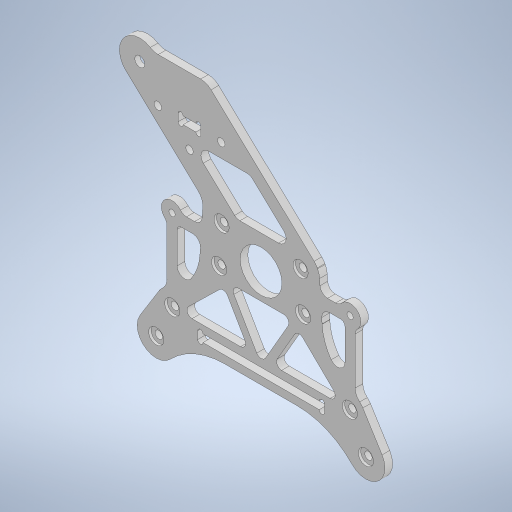
# Autodesk Inventor part: 内中間ユニット
Saved by Autodesk Inventor 2023 (Build 270158000, 158)
## iProperties
Created: 2022-06-23
Part Number: 内中間ユニット
Material: 一般
Document SubType Name: Modeling
Designer: muzho
Density: 1 g/cm^3
Appearance: 既定
Author: muzho
Autodesk Inventor part; units mm, degrees
ref_plane "YZ Plane" through (0, 0, 0) normal (1, 0, 0) x (0, 1, 0)
ref_plane "XZ Plane" through (0, 0, 0) normal (0, 1, 0) x (-1, 0, 0)
ref_plane "XY Plane" through (0, 0, 0) normal (0, 0, 1) x (1, 0, 0)
sketch "スケッチ1" plane through (0, 0, 0) normal (0, 0, 1) x (1, 0, 0)
  arc A0 (10.8616, 68.6715) -> (8.806, 69.4865) centre (8.806, 66.4865) ccw
  line L0 (10.8616, 68.6715) -> (23.2169, 57.0481)
  arc A1 (21.1613, 51.863) -> (23.2169, 57.0481) centre (21.1613, 54.863) ccw
  line L1 (21.1613, 51.863) -> (5.9002, 51.863)
  arc A2 (3.8446, 52.678) -> (5.9002, 51.863) centre (5.9002, 54.863) ccw
  line L2 (3.8446, 52.678) -> (-8.5107, 64.3014)
  arc A3 (-6.4551, 69.4865) -> (-8.5107, 64.3014) centre (-6.4551, 66.4865) ccw
  line L3 (-6.4551, 69.4865) -> (8.806, 69.4865)
  circle A4 centre (-1.4497, 74.9865) radius 1.5
  line L4 (35.1785, 52.6598) -> (-5.4497, 90.8816)
  arc A5 (-5.4497, 90.8816) -> (-9.561, 92.5115) centre (-9.561, 86.5115) ccw
  line L5 (-9.561, 92.5115) -> (-26.2964, 92.5115)
  arc A6 (-29.402, 93.3778) -> (-26.2964, 92.5115) centre (-26.2964, 98.5115) ccw
  arc A7 (-29.402, 93.3778) -> (-39.0547, 80.6665) centre (-33.5559, 86.5115) ccw
  line L6 (-39.0547, 80.6665) -> (-10.5496, 53.8498)
  arc A8 (-8.7348, 48.5407) -> (-10.5496, 53.8498) centre (-14.6609, 49.4798) ccw
  arc A9 (-8.7348, 48.5407) -> (-8.8114, 47.856) centre (-1.3025, 47.363) ccw
  line L7 (-8.9682, 45.4678) -> (-8.8114, 47.856)
  arc A10 (-11.9617, 42.6644) -> (-8.9682, 45.4678) centre (-11.9617, 45.6644) ccw
  line L8 (-15.1433, 42.6644) -> (-11.9617, 42.6644)
  arc A11 (-17.4955, 43.8023) -> (-15.1433, 42.6644) centre (-15.1433, 45.6644) ccw
  arc A12 (-17.4955, 43.8023) -> (-23.7588, 38.0868) centre (-20.8277, 41.1644) ccw
  arc A13 (-22.8277, 35.9144) -> (-23.7588, 38.0868) centre (-25.8277, 35.9144) ccw
  line L9 (-22.8277, 17.4431) -> (-22.8277, 35.9144)
  arc A14 (-24.6124, 13.614) -> (-22.8277, 17.4431) centre (-27.8277, 17.4431) ccw
  arc A15 (-24.6124, 13.614) -> (-25.8539, 12.1823) centre (-20.7379, 9) ccw
  line L10 (-33.4475, -0.0254) -> (-25.8539, 12.1823)
  arc A16 (-33.4475, -0.0254) -> (-21.6318, -9.2139) centre (-27.0578, -4) ccw
  arc A17 (0, 0) -> (-21.6318, -9.2139) centre (0, -30) ccw
  line L11 (28.5242, 0) -> (0, 0)
  arc A18 (50.156, -9.2139) -> (28.5242, 0) centre (28.5242, -30) ccw
  arc A19 (50.156, -9.2139) -> (61.9717, -0.0254) centre (55.582, -4) ccw
  line L12 (54.3781, 12.1823) -> (61.9717, -0.0254)
  arc A20 (54.3781, 12.1823) -> (53.1366, 13.614) centre (49.2621, 9) ccw
  arc A21 (51.3519, 17.4431) -> (53.1366, 13.614) centre (56.3519, 17.4431) ccw
  line L13 (51.3519, 35.9144) -> (51.3519, 17.4431)
  arc A22 (52.2829, 38.0868) -> (51.3519, 35.9144) centre (54.3519, 35.9144) ccw
  arc A23 (52.2829, 38.0868) -> (46.0197, 43.8023) centre (49.3519, 41.1644) ccw
  arc A24 (43.6675, 42.6644) -> (46.0197, 43.8023) centre (43.6675, 45.6644) ccw
  line L14 (40.4859, 42.6644) -> (43.6675, 42.6644)
  arc A25 (37.4924, 45.4678) -> (40.4859, 42.6644) centre (40.4859, 45.6644) ccw
  line L15 (37.3356, 47.856) -> (37.4924, 45.4678)
  arc A26 (37.3356, 47.856) -> (36.5452, 50.7523) centre (29.8267, 47.363) ccw
  line L16 (36.4243, 50.9921) -> (36.5452, 50.7523)
  arc A27 (36.4243, 50.9921) -> (35.1785, 52.6598) centre (31.0673, 48.2897) ccw
  circle A28 centre (-33.5559, 86.5115) radius 5.025
  arc A29 (-9.4497, 76.4865) -> (-11.4497, 76.4865) centre (-10.4497, 76.4865) ccw
  line L17 (-9.4497, 76.4865) -> (-9.4497, 73.4865)
  arc A30 (-11.4497, 73.4865) -> (-9.4497, 73.4865) centre (-10.4497, 73.4865) ccw
  line L18 (-11.4497, 73.4865) -> (-16.4497, 73.4865)
  arc A31 (-18.4497, 73.4865) -> (-16.4497, 73.4865) centre (-17.4497, 73.4865) ccw
  line L19 (-18.4497, 73.4865) -> (-18.4497, 76.4865)
  arc A32 (-16.4497, 76.4865) -> (-18.4497, 76.4865) centre (-17.4497, 76.4865) ccw
  line L20 (-16.4497, 76.4865) -> (-11.4497, 76.4865)
  circle A33 centre (-13.9497, 66.2015) radius 1.5
  circle A34 centre (-26.4497, 74.9865) radius 1.5
  line L21 (38.1817, 34.9678) -> (38.3215, 32.8383)
  arc A35 (41.1753, 38.1644) -> (38.1817, 34.9678) centre (41.1753, 35.1644) ccw
  line L22 (45.7302, 38.1644) -> (41.1753, 38.1644)
  arc A36 (47.3519, 36.5427) -> (45.7302, 38.1644) centre (45.7302, 36.5427) ccw
  line L23 (47.3519, 24.1122) -> (47.3519, 36.5427)
  arc A37 (41.8909, 22.3965) -> (47.3519, 24.1122) centre (44.3519, 24.1122) ccw
  arc A38 (38.3267, 32.7525) -> (41.8909, 22.3965) centre (58.2974, 33.8346) ccw
  arc A39 (38.3267, 32.7525) -> (38.3215, 32.8383) centre (30.8127, 32.3453) ccw
  arc A40 (5.2784, 28.5602) -> (3.5463, 25.5602) centre (5.2784, 26.5602) ccw
  line L24 (23.2458, 28.5602) -> (5.2784, 28.5602)
  arc A41 (24.9778, 25.5602) -> (23.2458, 28.5602) centre (23.2458, 26.5602) ccw
  line L25 (15.9941, 10) -> (24.9778, 25.5602)
  arc A42 (12.53, 10) -> (15.9941, 10) centre (14.2621, 11) ccw
  line L26 (3.5463, 25.5602) -> (12.53, 10)
  circle A43 centre (29.8267, 47.363) radius 3.025
  arc A44 (-14.363, 12.4314) -> (-12.9661, 9) centre (-12.9661, 11) ccw
  line L27 (-2.1172, 24.3817) -> (-14.363, 12.4314)
  arc A45 (1.0117, 23.9503) -> (-2.1172, 24.3817) centre (-0.7203, 22.9503) ccw
  line L28 (7.9112, 12) -> (1.0117, 23.9503)
  arc A46 (6.1792, 9) -> (7.9112, 12) centre (6.1792, 11) ccw
  line L29 (-12.9661, 9) -> (6.1792, 9)
  circle A47 centre (-2.2885, 32.3453) radius 3.025
  circle A48 centre (-20.7379, 9) radius 3.025
  circle A49 centre (-20.8277, 41.1644) radius 1.25
  line L30 (37.1621, 6) -> (-8.6379, 6)
  arc A50 (39.2621, 6) -> (37.1621, 6) centre (38.2121, 6) ccw
  line L31 (39.2621, 3) -> (39.2621, 6)
  arc A51 (37.1621, 3) -> (39.2621, 3) centre (38.2121, 3) ccw
  line L32 (-8.6379, 3) -> (37.1621, 3)
  arc A52 (-10.7379, 3) -> (-8.6379, 3) centre (-9.6879, 3) ccw
  line L33 (-10.7379, 6) -> (-10.7379, 3)
  arc A53 (-8.6379, 6) -> (-10.7379, 6) centre (-9.6879, 6) ccw
  circle A54 centre (-27.0578, -4) radius 3.025
  circle A55 centre (55.582, -4) radius 3.025
  circle A56 centre (49.2621, 9) radius 3.025
  circle A57 centre (49.3519, 41.1644) radius 1.25
  circle A58 centre (30.8127, 32.3453) radius 3.025
  arc A59 (30.6414, 24.3817) -> (27.5125, 23.9503) centre (29.2445, 22.9503) ccw
  line L34 (42.8871, 12.4314) -> (30.6414, 24.3817)
  arc A60 (41.4903, 9) -> (42.8871, 12.4314) centre (41.4903, 11) ccw
  line L35 (22.345, 9) -> (41.4903, 9)
  arc A61 (20.6129, 12) -> (22.345, 9) centre (22.345, 11) ccw
  line L36 (27.5125, 23.9503) -> (20.6129, 12)
  circle A62 centre (14.2621, 38.7999) radius 8.2397
  circle A63 centre (-1.3025, 47.363) radius 3.025
  arc A64 (-9.7973, 32.8383) -> (-9.8025, 32.7525) centre (-2.2885, 32.3453) ccw
  arc A65 (-13.3667, 22.3965) -> (-9.8025, 32.7525) centre (-29.7732, 33.8346) ccw
  arc A66 (-18.8277, 24.1122) -> (-13.3667, 22.3965) centre (-15.8277, 24.1122) ccw
  line L37 (-18.8277, 36.5427) -> (-18.8277, 24.1122)
  arc A67 (-17.206, 38.1644) -> (-18.8277, 36.5427) centre (-17.206, 36.5427) ccw
  line L38 (-12.6511, 38.1644) -> (-17.206, 38.1644)
  arc A68 (-9.6575, 34.9678) -> (-12.6511, 38.1644) centre (-12.6511, 35.1644) ccw
  line L39 (-9.7973, 32.8383) -> (-9.6575, 34.9678)
  circle A69 centre (-33.5559, 86.5115) radius 2
  circle A70 centre (-2.2885, 32.3453) radius 1.5
  circle A71 centre (-1.3025, 47.363) radius 1.5
  circle A72 centre (-20.7379, 9) radius 1.5
  circle A73 centre (-27.0578, -4) radius 1.5
  circle A74 centre (55.582, -4) radius 1.5
  circle A75 centre (49.2621, 9) radius 3.025
  circle A76 centre (30.8127, 32.3453) radius 1.5
  circle A77 centre (49.2621, 9) radius 1.5
  circle A78 centre (29.8267, 47.363) radius 1.5
  point P0 (14.2621, 9)
  constraints: 108 point on circle, 80 end point, 79 centre point, 15 horizontal, 8 vertical, 271 other
extrude "押し出し1" add sketch "スケッチ1" along normal blind 3 contours A27 L16 A26 L15 A25 L14 A24 A23 A22 L13 A21 A20 L12 A19 A18 L11 A17 A16 L10 A15 A14 L9 A13 A12 A11 L8 A10 L7 A9 A8 L6 A7 A6 L5 A5 L4
extrude "押し出し2" add sketch "スケッチ1" along normal blind 2 contours A43 | A47 | A48 | A54 | A55 | A56 | A58 | A63
sketch "スケッチ2" plane through (0, 0, 3) normal (0, 0, 1) x (-1, 0, 0)
  circle A0 centre (33.5559, -86.5115) radius 2 projected
  circle A1 centre (33.5559, -86.5115) radius 5.025 projected
  point P0 (0, 0)
extrude "押し出し3" add sketch "スケッチ2" against normal blind 2
